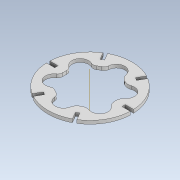
# Autodesk Inventor part: Ring_n2
Saved by Autodesk Inventor 2020 (Build 240168000, 168)
## iProperties
Created: 2020-09-11
Part Number: Ring_n2
Material: Generic
Document SubType Name: Modeling
Designer: Admin
Density: 1 g/cm^3
Appearance: Default
Author: Admin
Autodesk Inventor part; units mm, degrees
ref_plane "YZ Plane" through (0, 0, 0) normal (1, 0, 0) x (0, 1, 0)
ref_plane "XZ Plane" through (0, 0, 0) normal (0, 1, 0) x (-1, 0, 0)
ref_plane "XY Plane" through (0, 0, 0) normal (0, 0, 1) x (1, 0, 0)
sketch "Sketch1" plane through (0, 0, 0) normal (0, 1, 0) x (-1, 0, 0)
  circle A0 centre (0, 0) radius 25.325
  circle A1 centre (0, 0) radius 15.325
  dimension "d0" = 50.65
  dimension "d1" = 30.65
  constraints: 2 centre point, 2 coincident
  measures "d0" diameter of A0
  measures "d1" diameter of A1
extrude "Extrusion1" add sketch "Sketch1" along normal blind 2
sketch "Sketch2" plane through (0, 2, 0) normal (0, 1, 0) x (1, 0, 0)
  line L0 (-30.325, -1) -> (-20.325, -1)
  line L1 (-20.325, -1) -> (-20.325, 1)
  line L2 (-20.325, 1) -> (-30.325, 1)
  line L3 (-30.325, 1) -> (-30.325, -1)
  point P0 (0, 0)
  dimension "d8" = 20.325
  dimension "d9" = 1
  dimension "d10" = 2
  dimension "d11" = 10
  constraints: 8 end point, 2 parallel, 1 horizontal, 1 perpendicular
  measures "d8" distance from line of point (0, 0) L1
  measures "d9" distance from line of point (0, 0) L0
  measures "d10" distance of L2.end L0.start
  measures "d11" distance of L1.end L2.end
extrude "Extrusion2" cut sketch "Sketch2" against normal blind 2
pattern_circular "Circular Pattern1" count 6 over 360 about axis through (0, -10, 0) along (0, 1, 0) of "Extrusion2"
sketch "Sketch3" plane through (0, 2, 0) normal (0, 1, 0) x (1, 0, 0)
  circle A0 centre (-5.1962, -3) radius 10
  line L0 (-5.1962, -3) -> (0, 0) construction
  line L1 (-35.4273, 0) -> (35.4273, 0) projected
  dimension "d17" = 20
  dimension "d18" = 30
  dimension "d19" = 3
  constraints: 2 end point, 1 centre point
  measures "d17" diameter of A0
  measures "d18" angle of L0 L1
  measures "d19" distance from line of L1 L0.start
extrude "Extrusion3" cut sketch "Sketch3" against normal blind 2
pattern_circular "Circular Pattern2" count 6 over 360 about axis through (0, -10, 0) along (0, 1, 0) of "Extrusion3"
sketch "Sketch4" plane through (0, 2, 0) normal (0, 1, 0) x (1, 0, 0)
  circle A0 centre (13.8564, 8) radius 5
  line L0 (13.8564, 8) -> (0, 0) construction
  line L1 (-35.4273, 0) -> (35.4273, 0) projected
  dimension "d26" = 10
  dimension "d27" = 8
  dimension "d28" = 30
  constraints: 2 end point, 1 centre point
  measures "d26" diameter of A0
  measures "d27" vertical distance of L0.end L0.start
  measures "d28" angle of L1 L0
extrude "Extrusion4" cut sketch "Sketch4" against normal blind 2
pattern_circular "Circular Pattern3" count 6 over 360 about axis through (0, -10, 0) along (0, 1, 0) of "Extrusion4"
fillet "Fillet2" radius 3 12 edges at (-15.1945, 1, -3.1824) (-15.1649, 1, -2.2096) (-15.1649, 1, 2.2096) (-15.1945, 1, 3.1824) (-4.8412, 1, -14.75) (-5.6689, 1, -14.238) (-9.496, 1, -12.0284) (-10.3533, 1, -11.5676) (-4.8412, 1, 14.75) (-5.6689, 1, 14.238) (-10.3533, 1, 11.5676) (-9.496, 1, 12.0284)
fillet "Fillet3" radius 5 12 edges at (4.8412, 1, -14.75) (5.6689, 1, -14.238) (10.3533, 1, -11.5676) (9.496, 1, -12.0284) (15.1649, 1, -2.2096) (15.1945, 1, -3.1824) (15.1649, 1, 2.2096) (15.1945, 1, 3.1824) (10.3533, 1, 11.5676) (9.496, 1, 12.0284) (5.6689, 1, 14.238) (4.8412, 1, 14.75)
body "Solid1"
